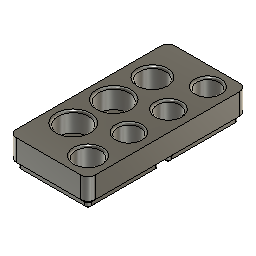
Gridfinity Hex Socket Holder 2x1 6-12 (Autodesk Fusion 360 design; units mm, degrees)
Autodesk Fusion 360 part; units mm, degrees
ref_plane "WorkPlane1" through (0, 0, 0) normal (0, 0, 1) x (1, 0, 0) in component "Gridfinity bin 2x1x2"
sketch "Sketch1" plane through (0, 0, 0) normal (0, 0, 1) x (1, 0, 0) in component "Gridfinity bin 2x1x2"
  line L0 (0, 0) -> (41.5, 0)
  line L1 (41.5, 0) -> (41.5, 41.5)
  line L2 (41.5, 41.5) -> (0, 41.5)
  line L3 (0, 41.5) -> (0, 0)
  dimension "d2" = 41.5
  dimension "d3" = 41.5
  constraint horizontal L0
  constraint vertical L1
  constraint horizontal L2
  constraint vertical L3
  constraint coincident L0.start L3
  constraint coincident L3.end L0
  measures "d2" horizontal distance of L0.start L0.end
  measures "d3" vertical distance of L0.end L1.end
extrude "Extrude1" add sketch "Sketch1" against normal blind 2.15 makes body 1 in component "Gridfinity bin 2x1x2"
fillet "Fillet1" radius 3.75 8 edges at (0, 0, -1.075) (41.5, 0, -1.075) (41.5, 0, -1.075) (41.5, 41.5, -1.075) (41.5, 41.5, -1.075) (0, 41.5, -1.075) (0, 41.5, -1.075) (0, 0, -1.075) on bodies 1 in component "Gridfinity bin 2x1x2"
chamfer "Chamfer1" distance 2.15 angle 45 8 edges at (1.0983, 40.4017, -2.15) (0, 20.75, -2.15) (1.0983, 1.0983, -2.15) (20.75, 0, -2.15) (40.4017, 1.0983, -2.15) (41.5, 20.75, -2.15) (40.4017, 40.4017, -2.15) (20.75, 41.5, -2.15) on bodies 1 in component "Gridfinity bin 2x1x2"
extrude "Extrude2" add 1 faces at (14.5499, 26.4167, -2.15) along direction (0, 0, -1) blind 2.6 on bodies 1 bodies 1 in component "Gridfinity bin 2x1x2"
chamfer "Chamfer2" distance 0.8 angle 45 8 edges at (2.6186, 38.8814, -4.75) (20.75, 39.35, -4.75) (38.8814, 38.8814, -4.75) (39.35, 20.75, -4.75) (38.8814, 2.6186, -4.75) (20.75, 2.15, -4.75) (2.6186, 2.6186, -4.75) (2.15, 20.75, -4.75) on bodies 1 in component "Gridfinity bin 2x1x2"
ref_plane "WorkPlane2" through (20.75, 20.75, -4.75) normal (0, 0, -1) x (-1, 0, 0) in component "Gridfinity bin 2x1x2"
sketch "Sketch2" plane through (20.75, 20.75, -4.75) normal (0, 0, -1) x (-1, 0, 0) in component "Gridfinity bin 2x1x2"
  circle A0 centre (13, -13) radius 3.25
  dimension "d13" = 6.5
  dimension "d14" = 13
  dimension "d15" = 13
  measures "d13" diameter of A0
  measures "d14" horizontal distance of origin A0.centre
  measures "d15" vertical distance of origin A0.centre
extrude "Extrude3" add sketch "Sketch2" against normal blind 2.4 separate body makes body 2 in component "Gridfinity bin 2x1x2"
pattern_linear "R-Pattern1" count 2 spacing 26 along (1, 0, 0) count 2 spacing 26 along (0, 1, 0) of bodies 2 makes body 3 at (30.5161, 7.4264, -3.95) makes body 4 at (4.5161, 33.4264, -3.95) makes body 5 at (30.5161, 33.4264, -3.95) in component "Gridfinity bin 2x1x2"
combine "Combine1" operation cut target body 1 tool bodies 2 3 4 5 2 in component "Gridfinity bin 2x1x2"
pattern_linear "R-Pattern2" count 1 spacing 42 along (1, 0, 0) count 2 spacing 42 along (0, 1, 0) of bodies 1 makes body 6 in component "Gridfinity bin 2x1x2"
sketch "Sketch3" plane through (0, 0, 0) normal (0, 0, 1) x (1, 0, 0) in component "Gridfinity bin 2x1x2"
  line L0 (0, 0) -> (41.5, 0)
  line L1 (41.5, 0) -> (41.5, 83.5)
  line L2 (41.5, 83.5) -> (0, 83.5)
  line L3 (0, 83.5) -> (0, 0)
  dimension "d26" = 41.5
  dimension "d27" = 83.5
  constraint horizontal L0
  constraint vertical L1
  constraint horizontal L2
  constraint vertical L3
  constraint coincident L0.start L3
  constraint coincident L3.end L0
  measures "d26" horizontal distance of L0.start L0.end
  measures "d27" vertical distance of L0.end L1.end
extrude "Extrude4" add sketch "Sketch3" along normal blind 11.21 separate body makes body 7 in component "Gridfinity bin 2x1x2"
fillet "Fillet2" radius 3.75 8 edges at (0, 83.5, 5.605) (41.5, 83.5, 5.605) (41.5, 83.5, 5.605) (41.5, 0, 5.605) (0, 0, 5.605) (0, 83.5, 5.605) (41.5, 0, 5.605) (0, 0, 5.605) on bodies 7 in component "Gridfinity bin 2x1x2"
combine "Combine2" operation add target body 7 tool bodies 1 6 1 in component "Gridfinity bin 2x1x2"
sketch "Sketch4" plane through (0, 0, 11.21) normal (0, 0, 1) x (-1, 0, 0) in component "Gridfinity bin 2x1x2"
  arc A0 (0, -3.75) -> (-3.75, 0) centre (-3.75, -3.75) ccw
  line L0 (-3.75, 0) -> (-37.75, 0)
  arc A1 (-37.75, 0) -> (-41.5, -3.75) centre (-37.75, -3.75) ccw
  line L1 (-41.5, -3.75) -> (-41.5, -79.75)
  arc A2 (-41.5, -79.75) -> (-37.75, -83.5) centre (-37.75, -79.75) ccw
  line L2 (-37.75, -83.5) -> (-3.75, -83.5)
  arc A3 (-3.75, -83.5) -> (0, -79.75) centre (-3.75, -79.75) ccw
  line L3 (0, -79.75) -> (0, -3.75)
  circle A4 centre (-12.025, -21.6583) radius 8.025
  circle A5 centre (-12.025, -42.9875) radius 8.025
  circle A6 centre (-12.025, -63.2917) radius 7
  circle A7 centre (-30.875, -10.625) radius 6.625
  circle A8 centre (-30.875, -32.0667) radius 6
  circle A9 centre (-30.875, -52.8833) radius 6
  circle A10 centre (-30.875, -73.6) radius 5.9
  line L4 (-30.875, -10.625) -> (-30.875, -73.6) construction
  line L5 (-30.875, -17.25) -> (-30.875, -26.0667)
  line L6 (-30.875, -38.0667) -> (-30.875, -46.8833)
  line L7 (-30.875, -58.8833) -> (-30.875, -67.7)
  line L8 (-12.025, -21.6583) -> (-12.025, -63.2917) construction
  line L9 (-30.875, -21.6583) -> (-12.025, -21.6583) construction
  line L10 (-30.875, -63.2917) -> (-12.025, -63.2917) construction
  line L11 (-12.025, -29.6833) -> (-12.025, -34.9625) construction
  line L12 (-12.025, -51.0125) -> (-12.025, -56.2917) construction
  dimension "d32" = 16.05
  dimension "d33" = 16.05
  dimension "d34" = 14
  dimension "d35" = 13.25
  dimension "d36" = 12
  dimension "d37" = 12
  dimension "d38" = 11.8
  dimension "d39" = 10.625
  dimension "d40" = 10.625
  dimension "d41" = 9.9
  dimension "d43" = 12.025
  constraint coincident A7.centre L4.start
  constraint vertical L4
  constraint coincident A10.centre L4
  constraint coincident A9.centre L4
  constraint coincident A8.centre L4
  constraint coincident A10.centre L4.end
  constraint coincident L4 L5.start
  constraint coincident A7 L5.start
  constraint coincident L4 L5.end
  constraint coincident A8 L5.end
  constraint coincident A8 L6.start
  constraint coincident L4 L6.start
  constraint coincident L4 L6.end
  constraint coincident A9 L6.end
  constraint coincident L4 L7.start
  constraint coincident A9 L7.start
  constraint coincident A10 L7.end
  constraint coincident L4 L7.end
  constraint equal L5 L6
  constraint equal L5 L7
  constraint coincident A4.centre L8.start
  constraint vertical L8
  constraint coincident A6.centre L8
  constraint coincident A5.centre L8
  constraint coincident A6.centre L8.end
  constraint midpoint L5 L9.start
  constraint perpendicular L8 L9
  constraint midpoint L7 L10.start
  constraint perpendicular L8 L10
  constraint coincident A4 L11.start
  constraint coincident L8 L11.start
  constraint coincident A5 L11.end
  constraint coincident L8 L11.end
  constraint coincident L8 L12.start
  constraint coincident A5 L12.start
  constraint coincident A6 L12.end
  constraint coincident L8 L12.end
  constraint equal L11 L12
  measures "d32" diameter of A4
  measures "d33" diameter of A5
  measures "d34" diameter of A6
  measures "d35" diameter of A7
  measures "d36" diameter of A8
  measures "d37" diameter of A9
  measures "d38" diameter of A10
  measures "d39" distance of L0 A7.centre
  measures "d40" distance of L1 A7.centre
  measures "d41" distance of L2 A10.centre
  measures "d43" distance of L3 A4.centre
extrude "Extrude5" cut sketch "Sketch4" against normal blind 10.3 contours A4 | A5 | A6 | A7 | A8 | A9 | A10 bodies 7 in component "Gridfinity bin 2x1x2"
fillet "Fillet3" radius 1 7 edges at (19.5069, 40.0855, 11.21) (19.5069, 18.7564, 11.21) (37.0517, 8.2293, 11.21) (36.469, 29.897, 11.21) (36.469, 50.7136, 11.21) (36.3757, 71.4665, 11.21) (18.5513, 60.7604, 11.21) on bodies 7 in component "Gridfinity bin 2x1x2"
component "Gridfinity bin 2x1x2" placed x (1, 0, 0) y (0, 1, 0) z (0, 0, 1) at (0, 0, 0)
equation "d4 = -( 2.15 mm )"
equation "d32 = 15.75 mm + 0.3 mm"
equation "d33 = 15.75 mm + 0.3 mm"
equation "d34 = 13.7 mm + 0.3 mm"
equation "d35 = 12.95 mm + 0.3 mm"
equation "d36 = 11.7 mm + 0.3 mm"
equation "d37 = 11.7 mm + 0.3 mm"
equation "d38 = 11.5 mm + 0.3 mm"
equation "d39 = ( 13.25 / 2 ) * 1 mm + WallOffset"
equation "d40 = ( 13.25 / 2 ) * 1 mm + WallOffset"
equation "d41 = ( 11.8 / 2 ) * 1 mm + WallOffset"
equation "WallOffset = 4 mm"
equation "d43 = ( 16.05 / 2 ) * 1 mm + WallOffset"
equation "d44 = -20.6 mm / 2"
named bodies: "base", "base (1)", "Gridfinity bin 2x1x2"
